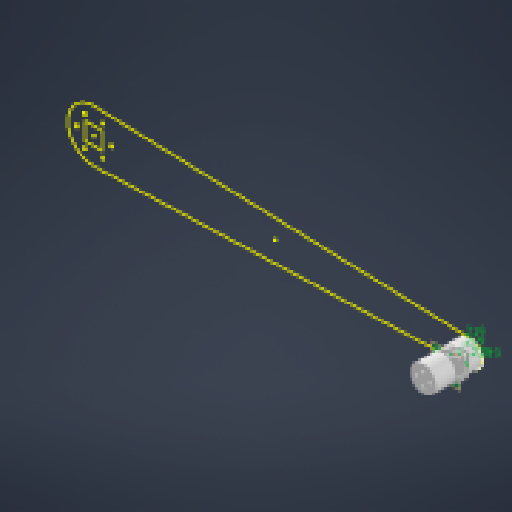
# Autodesk Inventor part: CarabinerThrowMount
Saved by Autodesk Inventor 2024.1 (Build 281209000, 209)
## iProperties
Created: 2023-10-16
Part Number: CarabinerThrowMount
Material: Generic
Document SubType Name: Modeling
Designer: Brandon
Density: 1 g/cm^3
Appearance: Default
Author: Brandon
Autodesk Inventor part; units mm, degrees
ref_plane "XZ Plane" through (0, 0, 0) normal (0, 1, 0) x (-1, 0, 0)
ref_plane "XY Plane" through (0, 0, 0) normal (0, 0, 1) x (1, 0, 0)
sketch "Sketch1" plane through (0, 0, 0) normal (0, 0, 1) x (1, 0, 0)
  line L0 (285.1848, -19.0386) -> (-264.1554, -38.0771) projected
  arc A0 (285.1848, -19.0386) -> (285.1848, 19.0386) centre (284.525, 0) ccw projected
  line L1 (-264.1554, 38.0771) -> (285.1848, 19.0386) projected
  arc A1 (-264.1554, 38.0771) -> (-264.1554, -38.0771) centre (-265.475, 0) ccw projected
  circle A2 centre (284.525, -9.525) radius 2 projected
  circle A3 centre (294.05, 0) radius 2 projected
  circle A4 centre (284.525, 9.525) radius 2 projected
  circle A5 centre (-290.875, 0) radius 2.1 projected
  circle A6 centre (-278.175, -21.997) radius 2.1 projected
  circle A7 centre (-252.775, -21.997) radius 2.1 projected
  circle A8 centre (-278.175, 21.997) radius 2.1 projected
  circle A9 centre (-252.775, 21.997) radius 2.1 projected
  line L2 (-252.775, -12.7) -> (-252.775, 12.7) projected
  line L3 (-278.175, -12.7) -> (-252.775, -12.7) projected
  line L4 (-278.175, 12.7) -> (-278.175, -12.7) projected
  line L5 (-252.775, 12.7) -> (-278.175, 12.7) projected
  circle A10 centre (-240.075, 0) radius 2.1 projected
  circle A11 centre (275, 0) radius 2 projected
  circle A12 centre (284.525, 0) radius 19.05
  circle A13 centre (275, 0) radius 2.7813
  circle A14 centre (284.525, 9.525) radius 2.7813
  circle A15 centre (294.05, 0) radius 2.7813
  circle A16 centre (284.525, -9.525) radius 2.7813
  point P0 (0, 0)
  dimension "d0" = 5.5626
  dimension "d1" = 5.5626
  dimension "d2" = 5.5626
  dimension "d3" = 5.5626
  constraints: 5 coincident, 4 centre point, 3 other
  measures "d0" diameter of A13
  measures "d1" diameter of A14
  measures "d2" diameter of A15
  measures "d3" diameter of A16
extrude "Extrusion1" add sketch "Sketch1" along normal blind 67.3 contours A12 A0 | A2 | A3 | A4 | A11 | A13 | A14 | A15 | A16
extrude "Extrusion3" cut sketch "Sketch1" along normal blind 19.05 contours A2 | A3 | A4 | A11
ref_plane "Work Plane1" through (284.525, 0, 33.65) normal (0, 0, -1) x (-1, 0, 0)
mirror "Mirror1" about plane through (284.525, 0, 33.65) normal (0, 0, -1) of "Extrusion3"
ref_plane "Work Plane4" through (284.525, 0, 33.65) normal (0, 0, -1) x (-1, 0, 0)
sketch "Sketch4" plane through (284.525, 0, 33.65) normal (0, 0, -1) x (-1, 0, 0)
  circle A0 centre (0, 0) radius 19.05 projected
  line L0 (0, -19.05) -> (15.24, -19.05)
  line L1 (19.05, -15.24) -> (19.05, 0)
  arc A1 (15.24, -19.05) -> (19.05, -15.24) centre (15.24, -15.24) ccw
  circle A2 centre (15.24, -15.24) radius 1.5
  circle A3 centre (-22.86, 0) radius 2
  line L2 (-22.86, 0) -> (-39.3578, 9.525)
  line L3 (0, 0) -> (-4.7364, 0)
  line L4 (-22.86, 0) -> (-22.86, 19.05)
  line L5 (-22.86, 0) -> (-8.2912, 20.8065)
  line L6 (-22.86, 0) -> (2.54, 0) construction
  line L7 (-22.86, 0) -> (-25.0738, 25.3033)
  arc A4 (-25.2699, 27.5448) -> (-24.8777, 23.0619) centre (-25.0738, 25.3033) ccw
  arc A5 (-9.5817, 18.9634) -> (-7.0006, 22.6496) centre (-8.2912, 20.8065) ccw
  arc A6 (-9.5817, 18.9634) -> (-24.8777, 23.0619) centre (-22.86, 0) ccw
  arc A7 (-7.0006, 22.6496) -> (-25.2699, 27.5448) centre (-22.86, 0) ccw
  circle A8 centre (-22.86, 0) radius 6.35
  circle A9 centre (-25.0738, 25.3033) radius 6.35
  circle A10 centre (-8.2912, 20.8065) radius 6.35
  line L8 (-10.5833, -15.8397) -> (-26.3878, -5.2799)
  line L9 (-29.1858, -0.5534) -> (-31.3996, 24.7499)
  line L10 (-6.6477, 26.9401) -> (-23.4303, 31.437)
  line L11 (10.5781, 15.8432) -> (-4.7651, 26.0875)
  line L12 (-17.6584, -3.6422) -> (-3.0895, 17.1643)
  point P0 (284.525, 0)
  point P1 (19.05, -7.62)
  point P2 (-18.4856, 4.6029)
  point P3 (-19.2178, 5.2016)
  point P4 (-17.3465, 7.8741)
  point P5 (-18.4856, -4.6029)
  point P6 (-29.5734, 3.876)
  point P7 (-28.3593, 3.175)
  dimension "d26" = 3.81
  dimension "d27" = 3
  dimension "d28" = 4
  dimension "d29" = 22.86
  dimension "d30" = 19.05
  dimension "d31" = 30
  dimension "d32" = 19.05
  dimension "d33" = 25.4
  dimension "d34" = 55
  dimension "d35" = 25.4
  dimension "d36" = 55
  dimension "d37" = 4.5
  dimension "d38" = 4.5
  dimension "d39" = 12.7
  dimension "d40" = 12.7
  dimension "d41" = 12.7
  dimension "d17" = 7.62
  dimension "d18" = 7.62
  constraints: 26 end point, 22 point on circle, 16 tangent, 10 centre point, 8 coincident, 3 horizontal, 1 equal length, 1 horizontal alignment, 1 midpoint, 1 perpendicular, 1 point on line, 1 vertical
  measures "d26" radius of A1
  measures "d27" diameter of A2
  measures "d28" diameter of A3
  measures "d29" distance of L2.start L3.start
  measures "d30" distance of L2.start L2.end
  measures "d31" angle of L3 L2
  measures "d32" distance of L2.start L4.end
  measures "d33" distance of L2.start L5.end
  measures "d34" angle of L6 L5
  measures "d35" distance of L2.start L7.end
  measures "d36" angle of L2 L7
  measures "d37" diameter of A4
  measures "d38" diameter of A5
  measures "d39" diameter of A8
  measures "d40" diameter of A9
  measures "d41" diameter of A10
extrude "Extrusion6" add sketch "Sketch4" along normal mid plane 10.16 contours A0 A8 L12 A10 | L1 A1 L0 A0 | A0 A10 L11 | A10 A0 | A0 A10 L5 A5 A7 | L8 A8 A0 | A10 L12 A8 A0 L5 | A0 L5 A10 | A10 A7 A9 L10 | A8 L2 A3 L5 A0 | A0 A8 | L5 A0 | A0 L5 A8 L7 A9 A6 A10 | A10 A6 L5 | A9 A7 A4 L7 | A8 L5 A0 | L9 L2 A8 | A9 L7 A8 L2 L9 | L5 A3 L4 A8 | A8 L7 A3 L2 | A9 L7 A6 | L4 A3 L7 A8
extrude "Extrusion7" cut sketch "Sketch4" along normal mid plane 6.35 contours A10 A0 | A0 A10 L5 A5 A7 | L8 A8 A0 | A10 L12 A8 A0 L5 | A0 L5 A10 | A10 A7 A9 L10 | A8 L2 A3 L5 A0 | A0 A8 | L5 A0 | A0 L5 A8 L7 A9 A6 A10 | A10 A6 L5 | A10 A6 A9 A7 | A7 A5 A6 A10 | A9 A7 A4 L7 | A8 L5 A0 | L9 L2 A8 | A9 A6 A4 A7 | A9 L7 A8 L2 L9 | L5 A3 L4 A8 | A8 L7 A3 L2 | A9 L7 A6 | L5 L4 A3 | A3 L2 L5 | L4 A3 L7 A8 | A3 L7 L2 | L4 L7 A3
fillet "Fillet1" radius 3.175 1 edges at (303.0106, -4.6029, 33.65)
fillet "Fillet2" radius 3.175 1 edges at (289.2901, 26.0875, 33.65)
body "Solid1"
